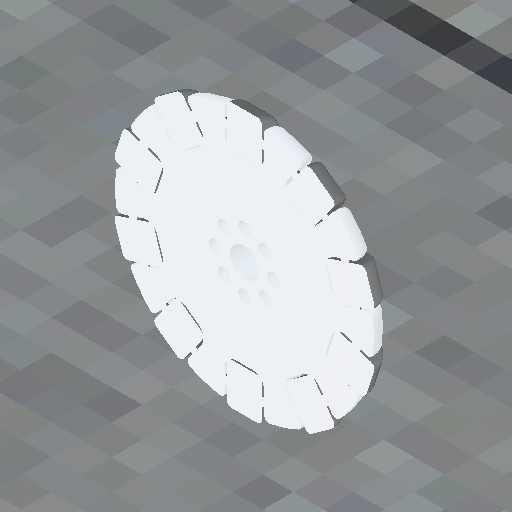
# Autodesk Inventor part: 3inch OmniWheel
Saved by Autodesk Inventor 2019 (Build 230136000, 136)
## iProperties
Created: 2012-11-03
Part Number: 3inch OmniWheel
Material: Generic
Document SubType Name: Modeling
Designer: Rob
Density: 1 g/cm^3
Mass: 19.784 g
Surface Area: 113.688 cm^2
Volume: 19.784 cm^3
Appearance: Snow
Author: Rob
Autodesk Inventor part; units mm, degrees
ref_plane "YZ Plane" through (0, 0, 0) normal (1, 0, 0) x (0, 1, 0)
ref_plane "XZ Plane" through (0, 0, 0) normal (0, 1, 0) x (-1, 0, 0)
ref_plane "XY Plane" through (0, 0, 0) normal (0, 0, 1) x (1, 0, 0)
sketch "Sketch1" plane through (0, 0, 0) normal (0, 0, 1) x (1, 0, 0)
  circle A0 centre (0, 0) radius 35.56
  dimension "d0" = 71.12
  constraints: 1 centre point, 1 coincident
  measures "d0" diameter of A0
extrude "Extrusion1" add sketch "Sketch1" along normal blind 10.16
fillet "Fillet1" radius 4.445 1 edges at (-35.56, 0, 10.16)
fillet "Fillet1" radius 4.445 1 edges at (-35.56, 0, 0)
sketch "Sketch2" plane through (0, 0, 10.16) normal (0, 0, 1) x (1, 0, 0)
  circle A0 centre (0, 0) radius 31.115 projected
  circle A1 centre (0, 0) radius 4.0005
  line L0 (0, 0) -> (0, 8.001)
  constraints: 2 end point, 1 centre point, 1 coincident
extrude "Extrusion2" cut sketch "Sketch2" against normal blind 12.7 contours A1
sketch "Sketch3" plane through (0, 0, 10.16) normal (0, 0, 1) x (1, 0, 0)
  circle A0 centre (0, 0) radius 31.115 projected
  line L0 (0, 0) -> (0, 8.001)
  constraints: 2 end point, 1 vertical
hole "Hole1" at (0, 8.001, 10.16) direction (0, 0, -1) diameter 3.4798 end through all
pattern_circular "Circular Pattern1" count 8 over 360 about axis through (0, 0, 10.16) along (0, 0, -1) of "Hole1"
sketch "Sketch4" plane through (0, 0, 10.16) normal (0, 0, 1) x (1, 0, 0)
  circle A0 centre (-5.6576, 5.6576) radius 1.7399 projected
  circle A1 centre (-8.001, 0) radius 1.7399 projected
  circle A2 centre (-5.6576, -5.6576) radius 1.7399 projected
  circle A3 centre (0, -8.001) radius 1.7399 projected
  circle A4 centre (5.6576, -5.6576) radius 1.7399 projected
  circle A5 centre (8.001, 0) radius 1.7399 projected
  circle A6 centre (5.6576, 5.6576) radius 1.7399 projected
  circle A7 centre (0, 8.001) radius 1.7399 projected
  circle A8 centre (0, 0) radius 4.0005 projected
  circle A9 centre (0, 0) radius 31.115 projected
  circle A10 centre (0, 0) radius 22.225
  dimension "d21" = 44.45
  constraints: 1 centre point, 1 coincident
  measures "d21" diameter of A10
extrude "Extrusion3" add sketch "Sketch4" along normal blind 1.27 contours A10
fillet "Fillet2" radius 1.27 1 edges at (-22.225, 0, 11.43)
sketch "Sketch5" plane through (0, 0, 0) normal (0, 0, -1) x (-1, 0, 0)
  circle A0 centre (5.6576, 5.6576) radius 1.7399 projected
  circle A1 centre (8.001, 0) radius 1.7399 projected
  circle A2 centre (5.6576, -5.6576) radius 1.7399 projected
  circle A3 centre (0, -8.001) radius 1.7399 projected
  circle A4 centre (-5.6576, -5.6576) radius 1.7399 projected
  circle A5 centre (-8.001, 0) radius 1.7399 projected
  circle A6 centre (-5.6576, 5.6576) radius 1.7399 projected
  circle A7 centre (0, 8.001) radius 1.7399 projected
  circle A8 centre (0, 0) radius 4.0005 projected
  circle A9 centre (0, 0) radius 31.115 projected
  circle A10 centre (0, 0) radius 22.225
  dimension "d25" = 44.45
  constraints: 1 centre point, 1 coincident
  measures "d25" diameter of A10
extrude "Extrusion4" add sketch "Sketch5" along normal blind 1.27 contours A10
fillet "Fillet3" radius 1.27 1 edges at (22.225, 0, -1.27)
sketch "Sketch6" plane through (0, 0, 10.16) normal (0, 0, 1) x (1, 0, 0)
  circle A0 centre (0, 0) radius 31.115 projected
  line L0 (5.4091, 35.1462) -> (5.4091, 27.6109)
  line L1 (2.2341, 24.4359) -> (0, 24.4359)
  line L2 (0, 24.4359) -> (-2.2341, 24.4359)
  line L3 (-5.4091, 27.6109) -> (-5.4091, 35.1462)
  arc A1 (5.4091, 35.1462) -> (-5.4091, 35.1462) centre (0, 0) ccw
  arc A2 (-5.4091, 27.6109) -> (-2.2341, 24.4359) centre (-2.2341, 27.6109) ccw
  arc A3 (2.2341, 24.4359) -> (5.4091, 27.6109) centre (2.2341, 27.6109) ccw
  dimension "d31" = 71.12
  dimension "d32" = 3.175
  constraints: 8 end point, 6 point on circle, 4 tangent, 3 centre point, 2 perpendicular, 1 coincident, 1 equal radius
  measures "d31" diameter of A1
  measures "d32" radius of A2
split body "Split1" sketch "Sketch6" result one side removed curves L0 A3 L1 L2 A2 L3 A1 removed pieces at (0.6797, 35.0042, 6.3361)
fillet "Fillet4" radius 1.27 18 edges at (-5.4091, 35.1462, 5.08) (-5.4091, 33.8172, 1.291) (-5.4091, 29.1261, 0) (-4.4791, 25.3659, 0) (-1.117, 24.4359, 0) (1.117, 24.4359, 0) (4.4791, 25.3659, 0) (5.4091, 29.1261, 0) (5.4091, 33.8172, 1.291) (5.4091, 35.1462, 5.08) (5.4091, 33.8172, 8.869) (5.4091, 29.1261, 10.16) (4.4791, 25.3659, 10.16) (-1.117, 24.4359, 10.16) (1.117, 24.4359, 10.16) (-4.4791, 25.3659, 10.16) (-5.4091, 29.1261, 10.16) (-5.4091, 33.8172, 8.869)
pattern_circular "Circular Pattern2" count 10 over 360 about axis through (0, 0, 10.16) along (0, 0, -1) of "Split1", "Fillet4"
sketch "Sketch7" plane through (-2.2341, 24.4359, 8.89) normal (0, 1, 0) x (1, 0, 0)
  line L0 (4.4682, 7.62) -> (4.4682, 0) projected
  line L1 (2.2341, 3.81) -> (-33.3259, 3.81)
  line L2 (2.2341, 3.81) -> (37.7941, 3.81)
  point P0 (2.2341, 8.89)
  dimension "d37" = 35.56
  dimension "d38" = 35.56
  constraints: 4 end point, 1 collinear, 1 perpendicular
  measures "d37" distance of L1.start L1.end
  measures "d38" distance of L1.start L2.end
split body "Split2" sketch "Sketch7" result one side removed curves L1 L2 removed pieces at (-5.26, -18.5397, 5.58)
sketch "Sketch8" plane through (-2.2341, 24.4359, 5.08) normal (0, 0, 1) x (1, 0, 0)
  line L0 (-3.175, 9.1973) -> (-3.175, 3.175) projected
  arc A0 (-28.7973, -7.0703) -> (-28.0815, -8.8983) centre (-27.6891, -7.6905) ccw projected
  arc A1 (-31.4245, -19.187) -> (-33.0781, -20.2452) centre (-31.817, -20.3949) ccw projected
  arc A2 (37.5463, -20.2452) -> (35.8927, -19.187) centre (36.2851, -20.3949) ccw projected
  line L1 (7.6432, 3.175) -> (7.6432, 9.1973) projected
  circle A3 centre (2.2341, -24.4359) radius 4.0005 projected
  line L2 (-2.5761, 6.1862) -> (7.0443, 6.1862)
  line L3 (-2.5761, 7.3744) -> (-2.5761, 10.6638)
  line L4 (-1.3061, 11.9338) -> (2.2341, 11.9338)
  line L5 (2.2341, 11.9338) -> (5.7743, 11.9338)
  line L6 (7.0443, 10.6638) -> (7.0443, 10.443)
  line L7 (7.0443, 10.443) -> (7.0443, 7.3744)
  arc A4 (-33.0781, -20.2452) -> (37.5463, -20.2452) centre (2.2341, -24.4359) ccw
  line L8 (-3.175, 6.1862) -> (7.6432, 6.1862)
  line L9 (7.6432, 6.1862) -> (7.6432, 7.3744)
  line L10 (-3.175, 7.3744) -> (-3.175, 6.1862)
  line L11 (7.6432, 7.3744) -> (7.0443, 7.3744)
  line L12 (-2.5761, 7.3744) -> (-3.175, 7.3744)
  arc A5 (-1.3061, 11.9338) -> (-2.5761, 10.6638) centre (-1.3061, 10.6638) ccw
  arc A6 (7.0443, 10.6638) -> (5.7743, 11.9338) centre (5.7743, 10.6638) ccw
  dimension "d39" = 1.27
  constraints: 22 end point, 9 point on circle, 4 parallel, 4 perpendicular, 4 tangent, 3 centre point, 1 coincident, 1 collinear, 1 equal radius, 1 horizontal, 1 midpoint, 1 point on line
  measures "d39" radius of A5
revolve "Revolution1" add sketch "Sketch8" angle 180 about axis through (-4.8102, 30.6221, 5.08) along (-1, 0, 0) contours L12 L3 A5 L4 L5 A6 L6 L7 L11 L1 L8 L2 L0
pattern_circular "Circular Pattern3" count 10 over 360 about axis through (0, 0, 10.16) along (0, 0, -1) of "Revolution1"
body "Solid1"
